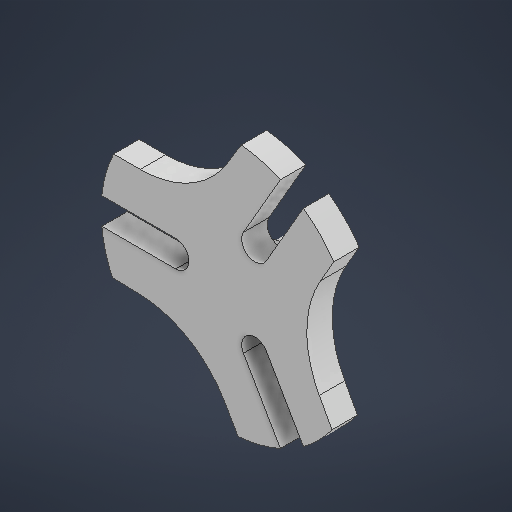
# Autodesk Inventor part: geniva2
Saved by Autodesk Inventor 2026.3 (Build 303398000, 398)
## iProperties
Created: 2026-04-30
Part Number: geniva2
Material: Generic
Document SubType Name: Modeling
Designer: frede
Density: 1 g/cm^3
Appearance: Default
Author: frede
Autodesk Inventor part; units mm, degrees
ref_plane "YZ Plane" through (0, 0, 0) normal (1, 0, 0) x (0, 1, 0)
ref_plane "XZ Plane" through (0, 0, 0) normal (0, 1, 0) x (-1, 0, 0)
ref_plane "XY Plane" through (0, 0, 0) normal (0, 0, 1) x (1, 0, 0)
sketch "Sketch1" plane through (0, 0, 0) normal (0, 0, 1) x (1, 0, 0)
  circle A0 centre (0, 0) radius 10.36
  arc A1 (-10.36, -2.6) -> (-10.36, 2.6) centre (-10.36, 0) ccw
  line L0 (-10.36, 2.6) -> (-24.8644, 2.6)
  line L1 (-10.36, -2.6) -> (-24.8644, -2.6)
  arc A2 (7.4317, -7.672) -> (2.9283, -10.272) centre (5.18, -8.972) ccw
  line L2 (2.9283, -10.272) -> (10.1806, -22.8332)
  line L3 (7.4317, -7.672) -> (14.6839, -20.2332)
  arc A3 (2.9283, 10.272) -> (7.4317, 7.672) centre (5.18, 8.972) ccw
  line L4 (7.4317, 7.672) -> (14.6839, 20.2332)
  line L5 (2.9283, 10.272) -> (10.1806, 22.8332)
  line L6 (-10.36, 2.6) -> (2.783, 9.9792)
  line L7 (0, 0) -> (-17.3112, 30.8327)
  arc A4 (-17.3112, 10.8327) -> (-0.2357, 20.4198) centre (-17.3112, 30.8327) ccw
  line L8 (-17.3112, 10.8327) -> (-22.5312, 10.8327)
  line L9 (-0.2357, 20.4198) -> (2.4821, 24.8765)
  line L10 (-17.5662, -10.414) -> (-22.7847, -10.2887)
  arc A5 (-0.7258, -20.4082) -> (-17.5662, -10.414) centre (-18.0463, -30.4082) ccw
  line L11 (-0.7258, -20.4082) -> (1.8842, -24.9289)
  line L12 (17.8019, -10.0058) -> (20.3026, -14.5878)
  arc A6 (18.0369, 9.5756) -> (17.8019, -10.0058) centre (35.3575, -0.4244) ccw
  line L13 (18.0369, 9.5756) -> (20.6469, 14.0962)
  arc A7 (20.6469, 14.0962) -> (14.6839, 20.2332) centre (0, 0) ccw
  arc A8 (10.1806, 22.8332) -> (2.4821, 24.8765) centre (0, 0) ccw
  arc A9 (-22.5312, 10.8327) -> (-24.8644, 2.6) centre (0, 0) ccw
  arc A10 (-24.8644, -2.6) -> (-22.7847, -10.2887) centre (0, 0) ccw
  arc A11 (1.8842, -24.9289) -> (10.1806, -22.8332) centre (0, 0) ccw
  arc A12 (14.6839, -20.2332) -> (20.3026, -14.5878) centre (0, 0) ccw
  point P0 (-24.0472, 10.8327)
  point P1 (3.2714, 26.1708)
  dimension "d1" = 20.72
  dimension "d2" = 5.2
  dimension "d5" = 360
  dimension "d7" = 35.36
  dimension "d8" = 40
  dimension "d11" = 360
  constraints: 28 end point, 27 point on circle, 13 centre point, 3 coincident, 3 horizontal, 3 tangent, 2 symmetric about line, 1 perpendicular, 50 other
  measures "d1" diameter of A0
  measures "d2" diameter of A1
  measures "d7" distance of L7.start L7.end
  measures "d8" diameter of A4
extrude "Extrusion1" add sketch "Sketch1" along normal blind 5 contours A0 A2 A1 L6 A3 | A0 A3 L4 A7 L13 A6 L12 A12 L3 A2 | L6 L7 A0 | A0 L7 A4 L9 A8 L5 A3 | A2 L2 A11 L11 A5 L10 A10 L1 A1 A0 | L7 L6 A0 | A0 L6 L0 A9 L8 A4 L7 | A0 A1 L6
sketch "Sketch2" plane through (0, 0, 0) normal (0, 0, -1) x (-1, 0, 0)
  circle A0 centre (0, 0) radius 2.5
  dimension "d15" = 5
  constraints: 1 centre point, 1 coincident
  measures "d15" diameter of A0
extrude "Extrusion2" add sketch "Sketch2" along normal blind 5
sketch "Sketch3" plane through (0, 0, -5) normal (0, 0, -1) x (-1, 0, 0)
  circle A0 centre (0, 0) radius 2.5 projected
  circle A1 centre (0, 0) radius 2
  dimension "d18" = 4
  constraints: 1 centre point, 1 coincident
  measures "d18" diameter of A1
extrude "Extrusion3" add sketch "Sketch3" along normal blind 5 contours A1
chamfer "Chamfer1" distance 0.25 angle 45 2 edges at (2, 0, -10) (2.5, 0, -5)
fillet "Fillet1" radius 2 1 edges at (2.5, 0, 0)
body "Solid1"
